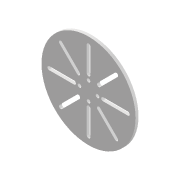
# Autodesk Inventor part: spool 4in outer plate
Saved by Autodesk Inventor 2020 (Build 240168000, 168)
## iProperties
Created: 2019-11-26
Part Number: spool 4in outer plate
Material: Generic
Document SubType Name: Modeling
Designer: ball
Density: 1 g/cm^3
Appearance: Default
Author: ball
Autodesk Inventor part; units mm, degrees
ref_plane "YZ Plane" through (0, 0, 0) normal (1, 0, 0) x (0, 1, 0)
ref_plane "XZ Plane" through (0, 0, 0) normal (0, 1, 0) x (-1, 0, 0)
ref_plane "XY Plane" through (0, 0, 0) normal (0, 0, 1) x (1, 0, 0)
sketch "Sketch1" plane through (0, 0, 0) normal (0, 0, 1) x (1, 0, 0)
  circle A0 centre (0, 0) radius 50.8
  circle A1 centre (9.779, 0) radius 1.778 construction
  circle A2 centre (0, 9.779) radius 1.778 construction
  circle A3 centre (-9.779, 0) radius 1.778 construction
  circle A4 centre (0, -9.779) radius 1.778 construction
  arc A5 (-9.6987, 7.1842) -> (-7.1842, 9.6987) centre (-8.4414, 8.4414) ccw construction
  circle A6 centre (9.6987, 0) radius 1.9304
  circle A7 centre (0, 9.779) radius 1.9304
  circle A8 centre (0, -9.779) radius 1.9304
  circle A9 centre (-9.779, 0) radius 1.9304
  circle A10 centre (0, 0) radius 42.545 construction
  circle A11 centre (0, 0) radius 15.5194 construction
  line L0 (0, -15.5194) -> (0, -42.545) construction
  line L1 (-1.9304, -15.5194) -> (-1.9304, -42.545)
  line L2 (1.9304, -42.545) -> (1.9304, -15.5194)
  arc A12 (1.9304, -15.5194) -> (-1.9304, -15.5194) centre (0, -15.5194) ccw
  arc A13 (-1.9304, -42.545) -> (1.9304, -42.545) centre (0, -42.545) ccw
  line L3 (31.4489, -28.7189) -> (12.3389, -9.6089)
  line L4 (9.6089, -12.3389) -> (28.7189, -31.4489)
  arc A14 (12.3389, -9.6089) -> (9.6089, -12.3389) centre (10.9739, -10.9739) ccw
  arc A15 (28.7189, -31.4489) -> (31.4489, -28.7189) centre (30.0839, -30.0839) ccw
  line L5 (42.545, 1.9304) -> (15.5194, 1.9304)
  line L6 (15.5194, -1.9304) -> (42.545, -1.9304)
  arc A16 (15.5194, 1.9304) -> (15.5194, -1.9304) centre (15.5194, 0) ccw
  arc A17 (42.545, -1.9304) -> (42.545, 1.9304) centre (42.545, 0) ccw
  line L7 (28.7189, 31.4489) -> (9.6089, 12.3389)
  line L8 (12.3389, 9.6089) -> (31.4489, 28.7189)
  arc A18 (9.6089, 12.3389) -> (12.3389, 9.6089) centre (10.9739, 10.9739) ccw
  arc A19 (31.4489, 28.7189) -> (28.7189, 31.4489) centre (30.0839, 30.0839) ccw
  line L9 (-1.9304, 42.545) -> (-1.9304, 15.5194)
  line L10 (1.9304, 15.5194) -> (1.9304, 42.545)
  arc A20 (-1.9304, 15.5194) -> (1.9304, 15.5194) centre (0, 15.5194) ccw
  arc A21 (1.9304, 42.545) -> (-1.9304, 42.545) centre (0, 42.545) ccw
  line L11 (-31.4489, 28.7189) -> (-12.3389, 9.6089)
  line L12 (-9.6089, 12.3389) -> (-28.7189, 31.4489)
  arc A22 (-12.3389, 9.6089) -> (-9.6089, 12.3389) centre (-10.9739, 10.9739) ccw
  arc A23 (-28.7189, 31.4489) -> (-31.4489, 28.7189) centre (-30.0839, 30.0839) ccw
  line L13 (-42.545, -1.9304) -> (-15.5194, -1.9304)
  line L14 (-15.5194, 1.9304) -> (-42.545, 1.9304)
  arc A24 (-15.5194, -1.9304) -> (-15.5194, 1.9304) centre (-15.5194, 0) ccw
  arc A25 (-42.545, 1.9304) -> (-42.545, -1.9304) centre (-42.545, 0) ccw
  line L15 (-28.7189, -31.4489) -> (-9.6089, -12.3389)
  line L16 (-12.3389, -9.6089) -> (-31.4489, -28.7189)
  arc A26 (-9.6089, -12.3389) -> (-12.3389, -9.6089) centre (-10.9739, -10.9739) ccw
  arc A27 (-31.4489, -28.7189) -> (-28.7189, -31.4489) centre (-30.0839, -30.0839) ccw
  circle A28 centre (0, 0) radius 6.35
  point P0 (0, -29.0322)
  dimension "d5" = 85.09
  dimension "d8" = 31.0388
  dimension "d0" = 101.6
  dimension "d1" = 3.8608
  dimension "d2" = 3.8608
  dimension "d3" = 3.8608
  dimension "d4" = 3.8608
  dimension "d9" = 3.8608
  dimension "d12" = 360
  dimension "d16" = 12.7
  constraints: 36 end point, 32 point on circle, 22 centre point, 7 coincident, 4 tangent, 2 vertical alignment, 1 midpoint, 1 parallel, 1 vertical, 85 other
  measures "d0" diameter of A0
  measures "d1" diameter of A6
  measures "d2" diameter of A7
  measures "d3" diameter of A8
  measures "d4" diameter of A9
  measures "d9" diameter of A13
  measures "d16" diameter of A28
extrude "Extrusion2" add sketch "Sketch1" along normal blind 3.175
body "Solid2"
